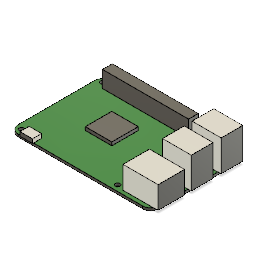
RPi (Autodesk Fusion 360 design; units mm, degrees)
Autodesk Fusion 360 part; units mm, degrees
sketch "Sketch1" plane through (0, 0, 0) normal (0, 1, 0) x (1, 0, 0)
  line L0 (11.7853, -3.8171) -> (86.7853, -3.8171)
  line L1 (91.7853, -8.8171) -> (91.7853, -54.8171)
  line L2 (86.7853, -59.8171) -> (11.7853, -59.8171)
  line L3 (6.7853, -54.8171) -> (6.7853, -8.8171)
  circle A0 centre (10.2853, -7.3171) radius 1.4
  circle A1 centre (10.2853, -56.3171) radius 1.4
  circle A2 centre (68.2853, -7.3171) radius 1.4
  circle A3 centre (68.2853, -56.3171) radius 1.4
  arc A4 (91.7853, -8.8171) -> (86.7853, -3.8171) centre (86.7853, -8.8171) ccw
  arc A5 (86.7853, -59.8171) -> (91.7853, -54.8171) centre (86.7853, -54.8171) ccw
  arc A6 (6.7853, -54.8171) -> (11.7853, -59.8171) centre (11.7853, -54.8171) ccw
  arc A7 (11.7853, -3.8171) -> (6.7853, -8.8171) centre (11.7853, -8.8171) ccw
  dimension "d1" = 85
  dimension "d2" = 56
  dimension "d3" = 58
  dimension "d4" = 2.8
  dimension "d5" = 3.5
  dimension "d6" = 3.5
  dimension "d7" = 49
  dimension "d8" = 5
  measures "d1" distance of origin
  measures "d2" distance of origin
  measures "d4" diameter of A0
  measures "d5" distance of L3
  measures "d6" distance of L0
  measures "d8" radius of A4
extrude "Extrude1" add sketch "Sketch1" along normal blind 1.6 makes body 1
copy_body "Body->Comp1" bodies 1 removing the originals makes body 2 in component "PCB"
sketch "Sketch1 (2)" plane through (0, 1.6, 0) normal (0, 1, 0) x (-1, 0, 0) in component "Component"
  circle A0 centre (-68.2853, 56.3171) radius 1.4
  circle A1 centre (-68.2853, 7.3171) radius 1.4
  circle A2 centre (-10.2853, 7.3171) radius 1.4
  circle A3 centre (-10.2853, 56.3171) radius 1.4
  arc A4 (-91.7853, 8.8171) -> (-86.7853, 3.8171) centre (-86.7853, 8.8171) ccw
  line L0 (-86.7853, 3.8171) -> (-11.7853, 3.8171)
  arc A5 (-11.7853, 3.8171) -> (-6.7853, 8.8171) centre (-11.7853, 8.8171) ccw
  line L1 (-6.7853, 8.8171) -> (-6.7853, 54.8171)
  arc A6 (-6.7853, 54.8171) -> (-11.7853, 59.8171) centre (-11.7853, 54.8171) ccw
  line L2 (-11.7853, 59.8171) -> (-86.7853, 59.8171)
  arc A7 (-86.7853, 59.8171) -> (-91.7853, 54.8171) centre (-86.7853, 54.8171) ccw
  line L3 (-91.7853, 54.8171) -> (-91.7853, 8.8171)
  line L4 (-72.7561, 41.6171) -> (-93.8853, 41.6171)
  line L5 (-93.8853, 41.6171) -> (-93.8853, 57.5171)
  line L6 (-93.8853, 57.5171) -> (-72.7561, 57.5171)
  line L7 (-72.7561, 57.5171) -> (-72.7561, 41.6171)
  dimension "d11" = 15.9
  dimension "d12" = 2.3
  dimension "d13" = 87.1
  measures "d12" distance of L2 L6
  measures "d13" distance of L1 L5
extrude "Extrude1'" add sketch "Sketch1 (2)" along normal blind 13.5 contours A7 L3 L4 L5 L6 | A7 L3 L4 L6 L7 bodies 2 in component "PCB"
sketch "Sketch2" plane through (0, 1.6, 0) normal (0, 1, 0) x (-1, 0, 0)
  line L0 (-72.7561, 41.6171) -> (-91.7853, 41.6171)
  line L1 (-91.7853, 41.6171) -> (-91.7853, 8.8171)
  arc A0 (-91.7853, 8.8171) -> (-86.7853, 3.8171) centre (-86.7853, 8.8171) ccw
  line L2 (-86.7853, 3.8171) -> (-11.7853, 3.8171)
  arc A1 (-11.7853, 3.8171) -> (-6.7853, 8.8171) centre (-11.7853, 8.8171) ccw
  line L3 (-6.7853, 8.8171) -> (-6.7853, 54.8171)
  arc A2 (-6.7853, 54.8171) -> (-11.7853, 59.8171) centre (-11.7853, 54.8171) ccw
  line L4 (-11.7853, 59.8171) -> (-86.7853, 59.8171)
  arc A3 (-86.7853, 59.8171) -> (-90.9936, 57.5171) centre (-86.7853, 54.8171) ccw
  line L5 (-90.9936, 57.5171) -> (-72.7561, 57.5171)
  line L6 (-72.7561, 57.5171) -> (-72.7561, 41.6171)
  circle A4 centre (-68.2853, 56.3171) radius 1.4
  circle A5 centre (-68.2853, 7.3171) radius 1.4
  circle A6 centre (-10.2853, 56.3171) radius 1.4
  circle A7 centre (-10.2853, 7.3171) radius 1.4
  line L7 (-13.5853, 55) -> (-21.0853, 55)
  line L8 (-21.0853, 55) -> (-21.0853, 60.4415)
  line L9 (-21.0853, 60.4415) -> (-13.5853, 60.4415)
  line L10 (-13.5853, 60.4415) -> (-13.5853, 55)
  dimension "d16" = 7.5
  dimension "d17" = 6.8
  measures "d16" distance of origin
  measures "d17" distance of L3
extrude "Extrude2" add sketch "Sketch2" along normal blind 2.5 contours L4 L8 L9 L10 | L4 L7 L8 L10 bodies 2 in component "PCB"
sketch "Sketch3" plane through (0, 1.6, 0) normal (0, 1, 0) x (-1, 0, 0)
  line L0 (-21.0853, 55) -> (-21.0853, 59.8171)
  line L1 (-21.0853, 59.8171) -> (-86.7853, 59.8171)
  arc A0 (-86.7853, 59.8171) -> (-90.9936, 57.5171) centre (-86.7853, 54.8171) ccw
  line L2 (-90.9936, 57.5171) -> (-72.7561, 57.5171)
  line L3 (-72.7561, 57.5171) -> (-72.7561, 41.6171)
  line L4 (-72.7561, 41.6171) -> (-91.7853, 41.6171)
  line L5 (-91.7853, 41.6171) -> (-91.7853, 8.8171)
  arc A1 (-91.7853, 8.8171) -> (-86.7853, 3.8171) centre (-86.7853, 8.8171) ccw
  line L6 (-86.7853, 3.8171) -> (-11.7853, 3.8171)
  arc A2 (-11.7853, 3.8171) -> (-6.7853, 8.8171) centre (-11.7853, 8.8171) ccw
  line L7 (-6.7853, 8.8171) -> (-6.7853, 54.8171)
  arc A3 (-6.7853, 54.8171) -> (-11.7853, 59.8171) centre (-11.7853, 54.8171) ccw
  line L8 (-11.7853, 59.8171) -> (-13.5853, 59.8171)
  line L9 (-13.5853, 59.8171) -> (-13.5853, 55)
  line L10 (-13.5853, 55) -> (-21.0853, 55)
  circle A4 centre (-68.2853, 56.3171) radius 1.4
  circle A5 centre (-68.2853, 7.3171) radius 1.4
  circle A6 centre (-10.2853, 56.3171) radius 1.4
  circle A7 centre (-10.2853, 7.3171) radius 1.4
  line L11 (-13.3683, 4.6362) -> (-65.3683, 4.6362)
  line L12 (-65.3683, 4.6362) -> (-65.3683, 10.6362)
  line L13 (-65.3683, 10.6362) -> (-13.3683, 10.6362)
  line L14 (-13.3683, 10.6362) -> (-13.3683, 4.6362)
  dimension "d20" = 52
  dimension "d21" = 6
  measures "d21" distance of L11 L13
extrude "Extrude3" add sketch "Sketch3" along normal blind 10 contours L11 L12 L13 L14 bodies 2 in component "PCB"
sketch "Sketch4" plane through (0, 1.6, 0) normal (0, 1, 0) x (-1, 0, 0)
  line L0 (-13.3683, 10.6362) -> (-13.3683, 4.6362)
  line L1 (-13.3683, 4.6362) -> (-65.3683, 4.6362)
  line L2 (-65.3683, 4.6362) -> (-65.3683, 10.6362)
  line L3 (-65.3683, 10.6362) -> (-13.3683, 10.6362)
  line L4 (-21.0853, 55) -> (-21.0853, 59.8171)
  line L5 (-21.0853, 59.8171) -> (-86.7853, 59.8171)
  arc A0 (-86.7853, 59.8171) -> (-90.9936, 57.5171) centre (-86.7853, 54.8171) ccw
  line L6 (-90.9936, 57.5171) -> (-72.7561, 57.5171)
  line L7 (-72.7561, 57.5171) -> (-72.7561, 41.6171)
  line L8 (-72.7561, 41.6171) -> (-91.7853, 41.6171)
  line L9 (-91.7853, 41.6171) -> (-91.7853, 8.8171)
  arc A1 (-91.7853, 8.8171) -> (-86.7853, 3.8171) centre (-86.7853, 8.8171) ccw
  line L10 (-86.7853, 3.8171) -> (-11.7853, 3.8171)
  arc A2 (-11.7853, 3.8171) -> (-6.7853, 8.8171) centre (-11.7853, 8.8171) ccw
  line L11 (-6.7853, 8.8171) -> (-6.7853, 54.8171)
  arc A3 (-6.7853, 54.8171) -> (-11.7853, 59.8171) centre (-11.7853, 54.8171) ccw
  line L12 (-11.7853, 59.8171) -> (-13.5853, 59.8171)
  line L13 (-13.5853, 59.8171) -> (-13.5853, 55)
  line L14 (-13.5853, 55) -> (-21.0853, 55)
  circle A4 centre (-68.2853, 56.3171) radius 1.4
  circle A5 centre (-68.2853, 7.3171) radius 1.4
  circle A6 centre (-10.2853, 56.3171) radius 1.4
  circle A7 centre (-10.2853, 7.3171) radius 1.4
  line L15 (-30.1471, 21.6994) -> (-46.1471, 21.6994)
  line L16 (-46.1471, 21.6994) -> (-46.1471, 37.6994)
  line L17 (-46.1471, 37.6994) -> (-30.1471, 37.6994)
  line L18 (-30.1471, 37.6994) -> (-30.1471, 21.6994)
  dimension "d24" = 16
  dimension "d25" = 16
extrude "Extrude4" add sketch "Sketch4" along normal blind 2 contours L15 L16 L17 L18 bodies 2 in component "PCB"
sketch "Sketch5" plane through (0, 1.6, 0) normal (0, 1, 0) x (-1, 0, 0)
  line L0 (-30.1471, 37.6994) -> (-30.1471, 21.6994)
  line L1 (-30.1471, 21.6994) -> (-46.1471, 21.6994)
  line L2 (-46.1471, 21.6994) -> (-46.1471, 37.6994)
  line L3 (-46.1471, 37.6994) -> (-30.1471, 37.6994)
  line L4 (-13.3683, 10.6362) -> (-13.3683, 4.6362)
  line L5 (-13.3683, 4.6362) -> (-65.3683, 4.6362)
  line L6 (-65.3683, 4.6362) -> (-65.3683, 10.6362)
  line L7 (-65.3683, 10.6362) -> (-13.3683, 10.6362)
  line L8 (-21.0853, 55) -> (-21.0853, 59.8171)
  line L9 (-21.0853, 59.8171) -> (-86.7853, 59.8171)
  arc A0 (-86.7853, 59.8171) -> (-90.9936, 57.5171) centre (-86.7853, 54.8171) ccw
  line L10 (-90.9936, 57.5171) -> (-72.7561, 57.5171)
  line L11 (-72.7561, 57.5171) -> (-72.7561, 41.6171)
  line L12 (-72.7561, 41.6171) -> (-91.7853, 41.6171)
  line L13 (-91.7853, 41.6171) -> (-91.7853, 8.8171)
  arc A1 (-91.7853, 8.8171) -> (-86.7853, 3.8171) centre (-86.7853, 8.8171) ccw
  line L14 (-86.7853, 3.8171) -> (-11.7853, 3.8171)
  arc A2 (-11.7853, 3.8171) -> (-6.7853, 8.8171) centre (-11.7853, 8.8171) ccw
  line L15 (-6.7853, 8.8171) -> (-6.7853, 54.8171)
  arc A3 (-6.7853, 54.8171) -> (-11.7853, 59.8171) centre (-11.7853, 54.8171) ccw
  line L16 (-11.7853, 59.8171) -> (-13.5853, 59.8171)
  line L17 (-13.5853, 59.8171) -> (-13.5853, 55)
  line L18 (-13.5853, 55) -> (-21.0853, 55)
  circle A4 centre (-68.2853, 56.3171) radius 1.4
  circle A5 centre (-68.2853, 7.3171) radius 1.4
  circle A6 centre (-10.2853, 56.3171) radius 1.4
  circle A7 centre (-10.2853, 7.3171) radius 1.4
  line L19 (-76.4643, 24.3171) -> (-93.7853, 24.3171)
  line L20 (-93.7853, 24.3171) -> (-93.7853, 37.4171)
  line L21 (-93.7853, 37.4171) -> (-76.4643, 37.4171)
  line L22 (-76.4643, 37.4171) -> (-76.4643, 24.3171)
  line L23 (-76.2496, 19.4171) -> (-93.7853, 19.4171)
  line L24 (-93.7853, 19.4171) -> (-93.7853, 6.3171)
  line L25 (-93.7853, 6.3171) -> (-76.2496, 6.3171)
  line L26 (-76.2496, 6.3171) -> (-76.2496, 19.4171)
  dimension "d28" = 13.1
  dimension "d29" = 4.2
  dimension "d30" = 2
  dimension "d31" = 13.1
  dimension "d32" = 4.9
  measures "d29" distance of L12 L21
  measures "d30" distance of L13 L20
  measures "d32" distance of L19 L23
extrude "Extrude5" add sketch "Sketch5" along normal blind 18.8 contours L13 L19 L21 L22 | L13 L19 L20 L21 | L13 A1 L23 L24 L25 | L13 A1 L23 L25 L26 bodies 2 in component "PCB"
component "Component" placed x (1, 0, 0) y (0, 1, 0) z (0, 0, 1) at (0, 0, 0)
component "PCB" placed x (1, 0, 0) y (0, 1, 0) z (0, 0, 1) at (0, 0, 0)
